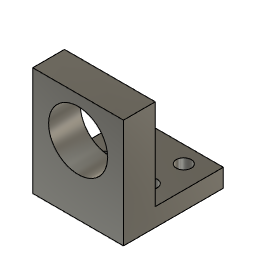
Rod Directional (Autodesk Fusion 360 design; units mm, degrees)
Autodesk Fusion 360 part; units mm, degrees
sketch "Sketch1" plane through (0, 0, 0) normal (0, 0, 1) x (1, 0, 0)
  line L0 (0, 0) -> (20, 0)
  line L1 (20, 0) -> (20, 15)
  line L2 (20, 15) -> (0, 15)
  line L3 (0, 15) -> (0, 0)
  dimension "d1" = 20
  dimension "d2" = 15
  constraint horizontal L0
  constraint vertical L1
  constraint horizontal L2
  constraint vertical L3
  constraint coincident L0.start L3.end
  measures "d1" distance of L0.start L0.end
  measures "d2" distance of L0.start L2.end
  measures "d5" distance of L0.start
extrude "Extrude1" add sketch "Sketch1" along normal blind 4
sketch "Sketch2" plane through (0, 0, 4) normal (0, 0, 1) x (-1, 0, 0)
  line L0 (0, -15) -> (0, 0)
  line L1 (0, 0) -> (-20, 0)
  line L2 (-20, 0) -> (-20, -15)
  line L3 (-20, -15) -> (0, -15)
  point P0 (-5, -11)
  point P1 (-15, -11)
  point P2 (-15, -3.5)
  point P3 (-5, -3.5)
  dimension "d5" = 10
  dimension "d6" = 10
  dimension "d7" = 5
  dimension "d8" = 5
  dimension "d9" = 4
  dimension "d10" = 7.5
  measures "d5" distance of P0 P1
  measures "d6" distance of P2 P3
  measures "d7" distance of L0 P0
  measures "d8" distance of L0 P3
  measures "d9" distance of L3 P0
  measures "d10" distance of P0 P3
hole "Hole1" at (5, 11, 4) at (15, 11, 4) at (15, 3.5, 4) at (5, 3.5, 4) direction (0, 0, -1) diameter 3.3 depth 11 tip angle 118
extrude "Extrude2" cut 1 faces at (13.3333, 15, 1.3333) along direction (0, -1, 0) blind 0.3
extrude "Extrude3" add 1 faces at (6.6667, 0, 1.3333) along direction (0, -1, 0) blind 0.3
extrude "Extrude4" add 1 faces at (6.6667, -0.3, 1.3333) along direction (0, -1, 0) blind 5
sketch "Sketch3" plane through (0, 0, 4) normal (0, 0, 1) x (-1, 0, 0)
  line L0 (-20, -14.7) -> (0, -14.7)
  line L1 (0, -14.7) -> (0, 5.3)
  line L2 (0, 5.3) -> (-20, 5.3)
  line L3 (-20, 5.3) -> (-20, -14.7)
  circle A0 centre (-5, -3.5) radius 1.65
  circle A1 centre (-15, -11) radius 1.65
  circle A2 centre (-5, -11) radius 1.65
  circle A3 centre (-15, -3.5) radius 1.65
  line L4 (0, 5.3) -> (-20, 5.3)
  line L5 (-20, 5.3) -> (-20, 0.3)
  line L6 (-20, 0.3) -> (0, 0.3)
  line L7 (0, 0.3) -> (0, 5.3)
  dimension "d20" = 5
  constraint horizontal L4
  constraint vertical L5
  constraint horizontal L6
  constraint vertical L7
  constraint coincident L1.end L2.start
  measures "d20" distance of L1.end L6.end
extrude "Extrude5" add sketch "Sketch3" along normal blind 20 contours L1 L2 L3 L4 L5 L6 L7
sketch "Sketch4" plane through (0, -0.3, 0) normal (0, 1, 0) x (-1, 0, 0)
  line L0 (-20, 4) -> (0, 4)
  line L1 (0, 4) -> (0, 24)
  line L2 (0, 24) -> (-20, 24)
  line L3 (-20, 24) -> (-20, 4)
  line L4 (0, 0) -> (-20, 0)
  point P0 (-10, 15.125)
  dimension "d23" = 15.125
  dimension "d24" = 10
  measures "d23" distance of P0 L4
  measures "d24" distance of L1 P0
hole "Hole2" at (10, -0.3, 15.125) direction (0, -1, 0) diameter 6.5 depth 11 tip angle 118
sketch "Sketch5" plane through (0, -0.3, 0) normal (0, 1, 0) x (-1, 0, 0)
  circle A0 centre (-10, 15.125) radius 3.25
  line L0 (-20, 4) -> (0, 4)
  line L1 (0, 4) -> (0, 24)
  line L2 (0, 24) -> (-20, 24)
  line L3 (-20, 24) -> (-20, 4)
  circle A1 centre (-10, 15.125) radius 3.75
  dimension "d28" = 7.5
  constraint concentric A0 A1
  measures "d28" diameter of A1
extrude "Extrude6" cut sketch "Sketch5" against normal blind 12.823 contours A1
sketch "Sketch6" plane through (0, -5.3, 0) normal (0, -1, 0) x (1, 0, 0)
  circle A0 centre (10, 15.125) radius 3.75
  line L0 (0, 0) -> (20, 0)
  line L1 (20, 0) -> (20, 24)
  line L2 (20, 24) -> (0, 24)
  line L3 (0, 24) -> (0, 0)
  circle A1 centre (10, 15.125) radius 6.5
  dimension "d31" = 13
  constraint concentric A0 A1
  measures "d31" diameter of A1
extrude "Extrude7" cut sketch "Sketch6" against normal blind 68.492 contours A1
extrude "Extrude8" add 1 faces at (9.8381, -5.3, 2.8811) along direction (0, -1, 0) blind 2
equation "d9 = 2.3 mm + 1.7 mm"
equation "d23 = 18.3 mm - ( 6.35 / 2 ) * 1 mm"
